Autodesk Fusion 360 part; units mm, degrees
(part 2 of 2)
sketch "Sketch11" plane through (0, 0, 0) normal (0, -1, 0) x (1, 0, 0)
  line L0 (51.4377, 4.5) -> (51.4377, 5)
  line L1 (51.4377, 5) -> (49.5623, 5)
  line L2 (49.5623, 5) -> (49.5623, 4.5)
  line L3 (49.5623, 4.5) -> (10, 4.5)
  line L4 (10, 4.5) -> (10, 0)
  line L5 (10, 0) -> (12, 0)
  line L6 (12, 0) -> (12, -22.5)
  line L7 (12, -22.5) -> (19, -22.5)
  line L8 (19, -22.5) -> (19, 0)
  line L9 (19, 0) -> (82, 0)
  line L10 (82, 0) -> (82, -22.5)
  line L11 (82, -22.5) -> (89, -22.5)
  line L12 (89, -22.5) -> (89, 0)
  line L13 (89, 0) -> (91, 0)
  line L14 (91, 0) -> (91, 4.5)
  line L15 (91, 4.5) -> (51.4377, 4.5)
  line L16 (10, 2.25) -> (91, 2.25) construction
  circle A0 centre (50.5, 2.25) radius 1.6
  circle A1 centre (13.5, 2.25) radius 1.6
  circle A2 centre (22.75, 2.25) radius 1.6
  circle A3 centre (32, 2.25) radius 1.6
  circle A4 centre (41.25, 2.25) radius 1.6
  circle A5 centre (59.75, 2.25) radius 1.6
  circle A6 centre (69, 2.25) radius 1.6
  circle A7 centre (78.25, 2.25) radius 1.6
  circle A8 centre (87.5, 2.25) radius 1.6
  dimension "d149" = 3.2
  dimension "d152" = 37
  dimension "d153" = 0
  constraint midpoint L4 L16.start
  constraint midpoint L14 L16.end
  constraint midpoint L16 A0.centre
  measures "d149" diameter of A0
extrude "Extrude8" cut sketch "Sketch11" against normal blind 5 contours A0 | A1 | A2 | A3 | A4 | A5 | A6 | A7 | A8 bodies 2 in component "chassis"
ref_plane "WorkPlane3" through (50.5, 80, -8.75) normal (0, -1, 0) x (1, 0, 0)
mirror "Mirror2" about plane through (50.5, 80, -8.75) normal (0, -1, 0) of "Extrude8" in component "chassis"
sketch "Sketch12" plane through (0, 0, 0) normal (0, 0, -1) x (1, 0, 0)
  line L0 (82, -118) -> (82, -134)
  line L1 (82, -134) -> (72, -134)
  line L2 (72, -134) -> (72, -118)
  line L3 (72, -118) -> (82, -118)
  line L4 (72, -26) -> (82, -26)
  line L5 (82, -26) -> (82, -42)
  line L6 (82, -42) -> (72, -42)
  line L7 (72, -42) -> (72, -26)
  line L8 (29, -134) -> (19, -134)
  line L9 (19, -134) -> (19, -118)
  line L10 (19, -118) -> (29, -118)
  line L11 (29, -118) -> (29, -134)
  line L12 (19, -26) -> (29, -26)
  line L13 (29, -26) -> (29, -42)
  line L14 (29, -42) -> (19, -42)
  line L15 (19, -42) -> (19, -26)
  circle A0 centre (91.9377, -2.6181) radius 1.6
  circle A1 centre (8.0795, -2.8802) radius 1.6
  circle A2 centre (89.5, -113.4279) radius 1.6
  circle A3 centre (12.1163, -133.9449) radius 1.6
  circle A4 centre (54.9377, -39.4681) radius 1.6
  circle A5 centre (31.1163, -78.4449) radius 1.6
  circle A6 centre (12.1163, -78.4449) radius 1.6
  circle A7 centre (45.0788, -2.6489) radius 1.6
  circle A8 centre (91.9377, -39.4681) radius 1.6
  circle A9 centre (8.3098, -39.7295) radius 1.6
  circle A10 centre (40.5, -113.4279) radius 1.6
  circle A11 centre (31.1163, -133.9449) radius 1.6
  circle A12 centre (89.5, -55.4279) radius 1.6
  circle A13 centre (40.5, -55.4279) radius 1.6
  circle A14 centre (54.9377, -2.6181) radius 1.6
  circle A15 centre (45.3091, -39.4982) radius 1.6
  arc A16 (15.4726, -155) -> (12.2734, -155) centre (13.873, -154.9634) ccw
  line L16 (15.4726, -155) -> (19, -155)
  line L17 (19, -155) -> (19, -160)
  line L18 (19, -160) -> (82, -160)
  line L19 (82, -160) -> (82, -156.4354)
  arc A17 (82.9726, -155) -> (82, -156.4354) centre (81.373, -154.9634) ccw
  line L20 (82.9726, -155) -> (87.2734, -155)
  arc A18 (89, -156.5583) -> (87.2734, -155) centre (88.873, -154.9634) ccw
  line L21 (89, -156.5583) -> (89, -160)
  line L22 (89, -160) -> (91, -160)
  arc A19 (91, -160) -> (101, -150) centre (91, -150) ccw
  line L23 (101, -150) -> (101, -10)
  arc A20 (101, -10) -> (91, 0) centre (91, -10) ccw
  line L24 (91, 0) -> (89, 0)
  line L25 (89, 0) -> (89, -5)
  line L26 (89, -5) -> (82, -5)
  line L27 (82, -5) -> (82, 0)
  line L28 (82, 0) -> (19, 0)
  line L29 (19, 0) -> (19, -5)
  line L30 (19, -5) -> (12, -5)
  line L31 (12, -5) -> (12, 0)
  line L32 (12, 0) -> (10, 0)
  arc A21 (10, 0) -> (0, -10) centre (10, -10) ccw
  line L33 (0, -10) -> (0, -150)
  arc A22 (0, -150) -> (10, -160) centre (10, -150) ccw
  line L34 (10, -160) -> (12, -160)
  line L35 (12, -160) -> (12, -155)
  line L36 (12, -155) -> (12.2734, -155)
  line L37 (50.0355, -61.6363) -> (56.0355, -65.1004)
  line L38 (56.0355, -65.1004) -> (56.0355, -72.0286)
  line L39 (56.0355, -72.0286) -> (50.0355, -75.4927)
  line L40 (50.0355, -75.4927) -> (44.0355, -72.0286)
  line L41 (44.0355, -72.0286) -> (44.0355, -65.1004)
  line L42 (44.0355, -65.1004) -> (50.0355, -61.6363)
  line L43 (50.0355, -59.4927) -> (44.0355, -56.0286)
  line L44 (44.0355, -56.0286) -> (44.0355, -52.5645)
  line L45 (44.0355, -52.5645) -> (56.0355, -52.5645)
  line L46 (56.0355, -52.5645) -> (56.0355, -56.0286)
  line L47 (56.0355, -56.0286) -> (50.0355, -59.4927)
  line L48 (50.0355, -77.6363) -> (56.0355, -81.1004)
  line L49 (56.0355, -81.1004) -> (56.0355, -88.0286)
  line L50 (56.0355, -88.0286) -> (50.0355, -91.4927)
  line L51 (50.0355, -91.4927) -> (44.0355, -88.0286)
  line L52 (44.0355, -88.0286) -> (44.0355, -81.1004)
  line L53 (44.0355, -81.1004) -> (50.0355, -77.6363)
  line L54 (50.0355, -109.6363) -> (56.0355, -113.1004)
  line L55 (56.0355, -113.1004) -> (56.0355, -120.0286)
  line L56 (56.0355, -120.0286) -> (50.0355, -123.4927)
  line L57 (50.0355, -123.4927) -> (44.0355, -120.0286)
  line L58 (44.0355, -120.0286) -> (44.0355, -113.1004)
  line L59 (44.0355, -113.1004) -> (50.0355, -109.6363)
  line L60 (78.3689, -93.6363) -> (84.3689, -97.1004)
  line L61 (84.3689, -97.1004) -> (84.3689, -104.0286)
  line L62 (84.3689, -104.0286) -> (78.3689, -107.4927)
  line L63 (78.3689, -107.4927) -> (72.3689, -104.0286)
  line L64 (72.3689, -104.0286) -> (72.3689, -97.1004)
  line L65 (72.3689, -97.1004) -> (78.3689, -93.6363)
  line L66 (60.6391, -137.4355) -> (58.2022, -136.0286)
  line L67 (58.2022, -136.0286) -> (58.2022, -129.1004)
  line L68 (58.2022, -129.1004) -> (64.2022, -125.6363)
  line L69 (64.2022, -125.6363) -> (70.2022, -129.1004)
  line L70 (70.2022, -129.1004) -> (70.2022, -136.0286)
  line L71 (70.2022, -136.0286) -> (67.7653, -137.4355)
  line L72 (67.7653, -137.4355) -> (60.6391, -137.4355)
  line L73 (13.5355, -104.0286) -> (9.2861, -106.482)
  line L74 (9.2861, -106.482) -> (9.2861, -94.647)
  line L75 (9.2861, -94.647) -> (13.5355, -97.1004)
  line L76 (13.5355, -97.1004) -> (13.5355, -104.0286)
  line L77 (29.8689, -40.0286) -> (29.8689, -33.1004)
  line L78 (29.8689, -33.1004) -> (35.8689, -29.6363)
  line L79 (35.8689, -29.6363) -> (41.8689, -33.1004)
  line L80 (41.8689, -33.1004) -> (41.8689, -40.0286)
  line L81 (41.8689, -40.0286) -> (39.3203, -41.5)
  line L82 (39.3203, -41.5) -> (32.4175, -41.5)
  line L83 (32.4175, -41.5) -> (29.8689, -40.0286)
  line L84 (58.2022, -33.1004) -> (64.2022, -29.6363)
  line L85 (64.2022, -29.6363) -> (70.2022, -33.1004)
  line L86 (70.2022, -33.1004) -> (70.2022, -40.0286)
  line L87 (70.2022, -40.0286) -> (67.6536, -41.5)
  line L88 (67.6536, -41.5) -> (60.7508, -41.5)
  line L89 (60.7508, -41.5) -> (58.2022, -40.0286)
  line L90 (58.2022, -40.0286) -> (58.2022, -33.1004)
  line L91 (64.2022, -11.4927) -> (58.2022, -8.0286)
  line L92 (58.2022, -8.0286) -> (58.2022, -2.0505)
  line L93 (58.2022, -2.0505) -> (70.2022, -2.0505)
  line L94 (70.2022, -2.0505) -> (70.2022, -8.0286)
  line L95 (70.2022, -8.0286) -> (64.2022, -11.4927)
  line L96 (13.5355, -17.1004) -> (13.5355, -24.0286)
  line L97 (13.5355, -24.0286) -> (7.5355, -27.4927)
  line L98 (7.5355, -27.4927) -> (7, -27.1835)
  line L99 (7, -27.1835) -> (7, -13.9455)
  line L100 (7, -13.9455) -> (7.5355, -13.6363)
  line L101 (7.5355, -13.6363) -> (13.5355, -17.1004)
  line L102 (56.0355, -17.1004) -> (56.0355, -24.0286)
  line L103 (56.0355, -24.0286) -> (53, -25.7811)
  line L104 (53, -25.7811) -> (53, -15.3478)
  line L105 (53, -15.3478) -> (56.0355, -17.1004)
  line L106 (21.7022, -77.6363) -> (27.7022, -81.1004)
  line L107 (27.7022, -81.1004) -> (27.7022, -88.0286)
  line L108 (27.7022, -88.0286) -> (21.7022, -91.4927)
  line L109 (21.7022, -91.4927) -> (15.7022, -88.0286)
  line L110 (15.7022, -88.0286) -> (15.7022, -81.1004)
  line L111 (15.7022, -81.1004) -> (21.7022, -77.6363)
  line L112 (29.8689, -120.0286) -> (29.8689, -113.1004)
  line L113 (29.8689, -113.1004) -> (34.3572, -110.509)
  line L114 (34.3572, -110.509) -> (34.3572, -122.6199)
  line L115 (34.3572, -122.6199) -> (29.8689, -120.0286)
  line L116 (86.5355, -65.1004) -> (92.5355, -61.6363)
  line L117 (92.5355, -61.6363) -> (92.5355, -75.4927)
  line L118 (92.5355, -75.4927) -> (86.5355, -72.0286)
  line L119 (86.5355, -72.0286) -> (86.5355, -65.1004)
  line L120 (64.2022, -93.6363) -> (70.2022, -97.1004)
  line L121 (70.2022, -97.1004) -> (70.2022, -104.0286)
  line L122 (70.2022, -104.0286) -> (64.2022, -107.4927)
  line L123 (64.2022, -107.4927) -> (58.2022, -104.0286)
  line L124 (58.2022, -104.0286) -> (58.2022, -97.1004)
  line L125 (58.2022, -97.1004) -> (64.2022, -93.6363)
  line L126 (41.8689, -72.0286) -> (37.6035, -74.4912)
  line L127 (37.6035, -74.4912) -> (37.5281, -62.5942)
  line L128 (37.5281, -62.5942) -> (41.8689, -65.1004)
  line L129 (41.8689, -65.1004) -> (41.8689, -72.0286)
  line L130 (64.2022, -77.6363) -> (70.2022, -81.1004)
  line L131 (70.2022, -81.1004) -> (70.2022, -88.0286)
  line L132 (70.2022, -88.0286) -> (64.2022, -91.4927)
  line L133 (64.2022, -91.4927) -> (58.2022, -88.0286)
  line L134 (58.2022, -88.0286) -> (58.2022, -81.1004)
  line L135 (58.2022, -81.1004) -> (64.2022, -77.6363)
  line L136 (78.3689, -59.4927) -> (72.3689, -56.0286)
  line L137 (72.3689, -56.0286) -> (72.3689, -52.5645)
  line L138 (72.3689, -52.5645) -> (84.3689, -52.5645)
  line L139 (84.3689, -52.5645) -> (84.3689, -56.0286)
  line L140 (84.3689, -56.0286) -> (78.3689, -59.4927)
  line L141 (64.2022, -61.6363) -> (70.2022, -65.1004)
  line L142 (70.2022, -65.1004) -> (70.2022, -72.0286)
  line L143 (70.2022, -72.0286) -> (64.2022, -75.4927)
  line L144 (64.2022, -75.4927) -> (58.2022, -72.0286)
  line L145 (58.2022, -72.0286) -> (58.2022, -65.1004)
  line L146 (58.2022, -65.1004) -> (64.2022, -61.6363)
  line L147 (78.3689, -61.6363) -> (84.3689, -65.1004)
  line L148 (84.3689, -65.1004) -> (84.3689, -72.0286)
  line L149 (84.3689, -72.0286) -> (78.3689, -75.4927)
  line L150 (78.3689, -75.4927) -> (72.3689, -72.0286)
  line L151 (72.3689, -72.0286) -> (72.3689, -65.1004)
  line L152 (72.3689, -65.1004) -> (78.3689, -61.6363)
  line L153 (41.8689, -88.0286) -> (37.7046, -90.4328)
  line L154 (37.7046, -90.4328) -> (37.6299, -78.653)
  line L155 (37.6299, -78.653) -> (41.8689, -81.1004)
  line L156 (41.8689, -81.1004) -> (41.8689, -88.0286)
  line L157 (50.0355, -93.6363) -> (56.0355, -97.1004)
  line L158 (56.0355, -97.1004) -> (56.0355, -104.0286)
  line L159 (56.0355, -104.0286) -> (50.0355, -107.4927)
  line L160 (50.0355, -107.4927) -> (44.0355, -104.0286)
  line L161 (44.0355, -104.0286) -> (44.0355, -97.1004)
  line L162 (44.0355, -97.1004) -> (50.0355, -93.6363)
  line L163 (86.5355, -97.1004) -> (92.5355, -93.6363)
  line L164 (92.5355, -93.6363) -> (92.5355, -107.4927)
  line L165 (92.5355, -107.4927) -> (86.5355, -104.0286)
  line L166 (86.5355, -104.0286) -> (86.5355, -97.1004)
  line L167 (46.4725, -137.4355) -> (44.0355, -136.0286)
  line L168 (44.0355, -136.0286) -> (44.0355, -129.1004)
  line L169 (44.0355, -129.1004) -> (50.0355, -125.6363)
  line L170 (50.0355, -125.6363) -> (56.0355, -129.1004)
  line L171 (56.0355, -129.1004) -> (56.0355, -136.0286)
  line L172 (56.0355, -136.0286) -> (53.5986, -137.4355)
  line L173 (53.5986, -137.4355) -> (46.4725, -137.4355)
  line L174 (13.5355, -120.0286) -> (9.2861, -122.482)
  line L175 (9.2861, -122.482) -> (9.2861, -110.647)
  line L176 (9.2861, -110.647) -> (13.5355, -113.1004)
  line L177 (13.5355, -113.1004) -> (13.5355, -120.0286)
  line L178 (35.8689, -13.6363) -> (41.8689, -17.1004)
  line L179 (41.8689, -17.1004) -> (41.8689, -24.0286)
  line L180 (41.8689, -24.0286) -> (35.8689, -27.4927)
  line L181 (35.8689, -27.4927) -> (29.8689, -24.0286)
  line L182 (29.8689, -24.0286) -> (29.8689, -17.1004)
  line L183 (29.8689, -17.1004) -> (35.8689, -13.6363)
  line L184 (86.5355, -24.0286) -> (86.5355, -17.1004)
  line L185 (86.5355, -17.1004) -> (92.5355, -13.6363)
  line L186 (92.5355, -13.6363) -> (94.007, -14.4858)
  line L187 (94.007, -14.4858) -> (94.007, -26.6431)
  line L188 (94.007, -26.6431) -> (92.5355, -27.4927)
  line L189 (92.5355, -27.4927) -> (86.5355, -24.0286)
  line L190 (35.8689, -11.4927) -> (29.8689, -8.0286)
  line L191 (29.8689, -8.0286) -> (29.8689, -2.0505)
  line L192 (29.8689, -2.0505) -> (41.8689, -2.0505)
  line L193 (41.8689, -2.0505) -> (41.8689, -8.0286)
  line L194 (41.8689, -8.0286) -> (35.8689, -11.4927)
  line L195 (64.2022, -13.6363) -> (70.2022, -17.1004)
  line L196 (70.2022, -17.1004) -> (70.2022, -24.0286)
  line L197 (70.2022, -24.0286) -> (64.2022, -27.4927)
  line L198 (64.2022, -27.4927) -> (58.2022, -24.0286)
  line L199 (58.2022, -24.0286) -> (58.2022, -17.1004)
  line L200 (58.2022, -17.1004) -> (64.2022, -13.6363)
  line L201 (44.0355, -17.1004) -> (47.9856, -14.8198)
  line L202 (47.9856, -14.8198) -> (47.9856, -26.3092)
  line L203 (47.9856, -26.3092) -> (44.0355, -24.0286)
  line L204 (44.0355, -24.0286) -> (44.0355, -17.1004)
  line L205 (21.7022, -93.6363) -> (27.7022, -97.1004)
  line L206 (27.7022, -97.1004) -> (27.7022, -104.0286)
  line L207 (27.7022, -104.0286) -> (21.7022, -107.4927)
  line L208 (21.7022, -107.4927) -> (15.7022, -104.0286)
  line L209 (15.7022, -104.0286) -> (15.7022, -97.1004)
  line L210 (15.7022, -97.1004) -> (21.7022, -93.6363)
  line L211 (29.8689, -97.1004) -> (34.3572, -94.509)
  line L212 (34.3572, -94.509) -> (34.3572, -106.6199)
  line L213 (34.3572, -106.6199) -> (29.8689, -104.0286)
  line L214 (29.8689, -104.0286) -> (29.8689, -97.1004)
  line L215 (86.5355, -81.1004) -> (92.5355, -77.6363)
  line L216 (92.5355, -77.6363) -> (92.5355, -91.4927)
  line L217 (92.5355, -91.4927) -> (86.5355, -88.0286)
  line L218 (86.5355, -88.0286) -> (86.5355, -81.1004)
  line L219 (64.2022, -109.6363) -> (70.2022, -113.1004)
  line L220 (70.2022, -113.1004) -> (70.2022, -120.0286)
  line L221 (70.2022, -120.0286) -> (64.2022, -123.4927)
  line L222 (64.2022, -123.4927) -> (58.2022, -120.0286)
  line L223 (58.2022, -120.0286) -> (58.2022, -113.1004)
  line L224 (58.2022, -113.1004) -> (64.2022, -109.6363)
  line L225 (41.8689, -104.0286) -> (37.8058, -106.3744)
  line L226 (37.8058, -106.3744) -> (37.7318, -94.7118)
  line L227 (37.7318, -94.7118) -> (41.8689, -97.1004)
  line L228 (41.8689, -97.1004) -> (41.8689, -104.0286)
  line L229 (78.3689, -77.6363) -> (84.3689, -81.1004)
  line L230 (84.3689, -81.1004) -> (84.3689, -88.0286)
  line L231 (84.3689, -88.0286) -> (78.3689, -91.4927)
  line L232 (78.3689, -91.4927) -> (72.3689, -88.0286)
  line L233 (72.3689, -88.0286) -> (72.3689, -81.1004)
  line L234 (72.3689, -81.1004) -> (78.3689, -77.6363)
  line L235 (64.2022, -59.4927) -> (58.2022, -56.0286)
  line L236 (58.2022, -56.0286) -> (58.2022, -52.5645)
  line L237 (58.2022, -52.5645) -> (70.2022, -52.5645)
  line L238 (70.2022, -52.5645) -> (70.2022, -56.0286)
  line L239 (70.2022, -56.0286) -> (64.2022, -59.4927)
  circle A23 centre (6.373, -148.9634) radius 1.6
  circle A24 centre (13.873, -142.9634) radius 1.6
  circle A25 centre (28.873, -154.9634) radius 1.6
  circle A26 centre (36.373, -148.9634) radius 1.6
  circle A27 centre (43.873, -142.9634) radius 1.6
  circle A28 centre (58.873, -154.9634) radius 1.6
  circle A29 centre (66.373, -148.9634) radius 1.6
  circle A30 centre (73.873, -142.9634) radius 1.6
  circle A31 centre (96.373, -142.9634) radius 1.6
  circle A32 centre (88.873, -148.9634) radius 1.6
  circle A33 centre (66.373, -142.9634) radius 1.6
  circle A34 centre (58.873, -148.9634) radius 1.6
  circle A35 centre (51.373, -154.9634) radius 1.6
  circle A36 centre (36.373, -142.9634) radius 1.6
  circle A37 centre (28.873, -148.9634) radius 1.6
  circle A38 centre (21.373, -154.9634) radius 1.6
  circle A39 centre (6.373, -142.9634) radius 1.6
  circle A40 centre (13.873, -148.9634) radius 1.6
  circle A41 centre (21.373, -142.9634) radius 1.6
  circle A42 centre (36.373, -154.9634) radius 1.6
  circle A43 centre (43.873, -148.9634) radius 1.6
  circle A44 centre (51.373, -142.9634) radius 1.6
  circle A45 centre (66.373, -154.9634) radius 1.6
  circle A46 centre (73.873, -148.9634) radius 1.6
  circle A47 centre (81.373, -142.9634) radius 1.6
  circle A48 centre (96.373, -148.9634) radius 1.6
  circle A49 centre (88.873, -142.9634) radius 1.6
  circle A50 centre (81.373, -148.9634) radius 1.6
  circle A51 centre (73.873, -154.9634) radius 1.6
  circle A52 centre (58.873, -142.9634) radius 1.6
  circle A53 centre (51.373, -148.9634) radius 1.6
  circle A54 centre (43.873, -154.9634) radius 1.6
  circle A55 centre (28.873, -142.9634) radius 1.6
  circle A56 centre (21.373, -148.9634) radius 1.6
  line L240 (50.5, -160) -> (50.5, 0) construction
  line L241 (19, -26) -> (19, -134) construction
  line L242 (15, -50) -> (25, -50)
  line L243 (25, -50) -> (25, -75)
  line L244 (25, -75) -> (15, -75)
  line L245 (15, -75) -> (15, -50)
  line L246 (86, -75) -> (86, -50)
  line L247 (86, -50) -> (76, -50)
  line L248 (76, -50) -> (76, -75)
  line L249 (76, -75) -> (86, -75)
  constraint midpoint L18 L240.start
  constraint midpoint L28 L240.end
  constraint coincident L12.start L15.end
  constraint coincident L8.end L9.start
  constraint horizontal L242
  constraint vertical L243
  constraint horizontal L244
  constraint vertical L245
  constraint symmetric L240 L242.start L246.end
  constraint symmetric L240 L242.end L247.end
  constraint symmetric L240 L243.end L248.end
  constraint symmetric L240 L244.end L246.start
sketch "Sketch13" plane through (86, 0, 0) normal (1, 0, 0) x (0, 1, 0)
  line L0 (75, 0) -> (50, 0)
  line L1 (50, 0) -> (50, -10)
  line L2 (50, -10) -> (75, -10)
  line L3 (75, -10) -> (75, 0)
  line L4 (72, -7) -> (53, -7)
  line L5 (53, -7) -> (53, -1)
  line L6 (53, -1) -> (72, -1)
  line L7 (72, -1) -> (72, -7)
  constraint horizontal L4
  constraint vertical L5
  constraint horizontal L6
  constraint vertical L7
component "chassis" placed x (1, 0, 0) y (0, 1, 0) z (0, 0, 1) at (0, 0, 0)
